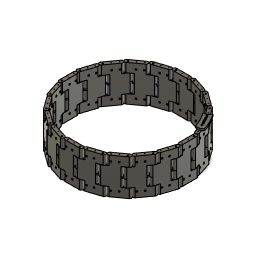
CAT_Wheel_Part v7 (Autodesk Fusion 360 design; units mm, degrees)
Autodesk Fusion 360 part; units mm, degrees
sketch "R_Part" plane through (0, 0, 0) normal (0, 1, 0) x (1, 0, 0)
  line L0 (75, 100) -> (0, 100)
  line L1 (0, 100) -> (0, 0)
  line L2 (150, 100) -> (150, 150)
  line L3 (150, 150) -> (75, 150)
  line L4 (75, 150) -> (75, 100)
  line L5 (150.000002, 100) -> (150.000002, 0)
  line L6 (150.000002, 0) -> (75, 0)
  line L7 (0, -50.000001) -> (75, -50)
  line L8 (75, -50) -> (75, 0)
  line L9 (0, 0) -> (0, -50.000001)
  dimension "d1" = 75
  dimension "d2" = 100
  dimension "d3" = 75
  dimension "d4" = 50
  dimension "d5" = 50
  dimension "d6" = 75.000002
  dimension "d7" = 150.000002
  constraint horizontal L0
  constraint vertical L1
  constraint coincident L1.end L9.start
  constraint vertical L2
  constraint horizontal L3
  constraint vertical L4
  constraint vertical L5
  constraint horizontal L6
  constraint horizontal L7
  constraint vertical L8
  constraint perpendicular L7 L9
  measures "d1" distance of L1.end L6.end
  measures "d2" distance of L1.end L0.end
  measures "d3" distance of L0.start L2.start
  measures "d4" distance of L0.start L3.end
  measures "d5" distance of L6.end L7.end
  measures "d7" distance of L1 L5
extrude "Extrude1" add sketch "R_Part" along normal blind 50 contours L0 L1 L2 L3 L4 L5 L6 L7 L8 L9 picked at (125.000001, 33.333333) makes body 1
extrude "Extrude2" cut 1 faces at (125.000001, 50, -33.333333) along direction (0, -1, 0) blind 20 on bodies 1 bodies 1
sketch "L_Part" plane through (0, 0, 0) normal (0, 1, 0) x (1, 0, 0)
  line L0 (-75, 0) -> (-150, 0)
  line L1 (-150, 0) -> (-150, 100)
  line L2 (-75, 100) -> (0, 100)
  line L3 (0, 100) -> (0, 0)
  line L4 (-75, 100) -> (-75, 150)
  line L5 (-75, 150) -> (-150, 150)
  line L6 (-150, 150) -> (-150, 100)
  line L7 (-75, 0) -> (-75, -50)
  line L8 (-75, -50) -> (0, -50)
  line L9 (0, -50) -> (0, 0)
  dimension "d13" = 150
  dimension "d14" = 100
  dimension "d15" = 75
  dimension "d16" = 50
  dimension "d17" = 75
  dimension "d18" = 50
  constraint horizontal L0
  constraint vertical L1
  constraint horizontal L2
  constraint vertical L3
  constraint coincident L3.end L9.end
  constraint vertical L4
  constraint horizontal L5
  constraint vertical L6
  constraint vertical L7
  constraint horizontal L8
  constraint vertical L9
  measures "d13" distance of L3.end L0.end
  measures "d14" distance of L3.end L2.end
  measures "d15" distance of L1.end L2.start
  measures "d16" distance of L1.end L5.end
  measures "d17" distance of L3.end L0.start
  measures "d18" distance of L3.end L8.end
sketch "Sketch3" plane through (0, 0, 50.000001) normal (0, 0, 1) x (1, 0, 0)
  line L0 (75, 30) -> (0, 30)
  line L1 (0, 30) -> (0, 0)
  line L2 (0, 0) -> (75, 0)
  line L3 (75, 0) -> (75, 30)
  line L4 (0, 0) -> (-10, 0)
  line L5 (-10, 0) -> (-10, 15)
  line L6 (-10, 15) -> (0, 15)
  line L7 (0, 15) -> (0, 0)
  line L8 (0, 15) -> (10, 15)
  line L9 (10, 15) -> (10, 30)
  line L10 (10, 30) -> (0, 30)
  line L11 (0, 30) -> (0, 15)
  dimension "d21" = 15
  dimension "d22" = 10
  dimension "d23" = 10
  constraint horizontal L4
  constraint vertical L5
  constraint horizontal L6
  constraint vertical L7
  constraint coincident L1.end L2.start
  constraint horizontal L8
  constraint vertical L9
  constraint horizontal L10
  constraint vertical L11
  measures "d21" distance of L1.end L6.end
  measures "d22" distance of L1.end L4.end
  measures "d23" distance of L6.end L8.end
extrude "Extrude4" add sketch "Sketch3" against normal blind 150 contours L1 L4 L5 L6 L7 picked at (-3.333334, 10) bodies 1
extrude "Extrude5" cut sketch "Sketch3" against normal blind 150 contours L0 L1 L8 L9 L10 L11 picked at (3.333333, 25) bodies 1
sketch "Sketch4" plane through (75, 0, 0) normal (1, 0, 0) x (0, 0, -1)
  line L0 (0, 30) -> (-50, 30)
  line L1 (-50, 30) -> (-50, 0)
  line L2 (-50, 0) -> (0, 0)
  line L3 (0, 0) -> (0, 30)
  circle A0 centre (-25, 15) radius 2.75
  dimension "d28" = 5.5
  measures "d28" diameter of A0
extrude "Extrude6" cut sketch "Sketch4" against normal blind 95 contours A0 picked at (-25.720575, 16.369678) bodies 1
sketch "Sketch5" plane through (75, 0, 0) normal (-1, 0, 0) x (0, 0, 1)
  line L0 (-100, 30) -> (-150, 30)
  line L1 (-150, 30) -> (-150, 0)
  line L2 (-150, 0) -> (-100, 0)
  line L3 (-100, 0) -> (-100, 30)
  circle A0 centre (-125, 15) radius 2.75
  dimension "d31" = 5.5
  measures "d31" diameter of A0
extrude "Extrude7" cut sketch "Sketch5" against normal blind 76 contours A0 picked at (-125.470371, 15.87372) bodies 1
sketch "Sketch6" plane through (150, 0, 0) normal (1, 0, 0) x (0, 0, -1)
  circle A0 centre (125, 15) radius 2.75
  line L0 (150, 30) -> (0, 30)
  line L1 (0, 30) -> (0, 0)
  line L2 (0, 0) -> (150, 0)
  line L3 (150, 0) -> (150, 30)
  line L4 (129.2, 17.424871) -> (125, 19.849742)
  line L5 (125, 19.849742) -> (120.8, 17.424871)
  line L6 (120.8, 17.424871) -> (120.8, 12.575129)
  line L7 (120.8, 12.575129) -> (125, 10.150258)
  line L8 (125, 10.150258) -> (129.2, 12.575129)
  line L9 (129.2, 12.575129) -> (129.2, 17.424871)
  point P0 (125, 15)
  dimension "d34" = 4.2
  constraint coincident P0 A0.centre
  measures "d34" distance of P0 L9
extrude "Extrude8" cut sketch "Sketch6" against normal blind 4.5 contours L4 L5 L6 L7 L8 L9 picked at (121.283333, 15) bodies 1
sketch "Sketch7" plane through (150, 0, 0) normal (1, 0, 0) x (0, 0, -1)
  line L0 (125, 19.849742) -> (129.2, 17.424871)
  line L1 (129.2, 17.424871) -> (129.2, 12.575129)
  line L2 (129.2, 12.575129) -> (125, 10.150258)
  line L3 (125, 10.150258) -> (120.8, 12.575129)
  line L4 (120.8, 12.575129) -> (120.8, 17.424871)
  line L5 (120.8, 17.424871) -> (125, 19.849742)
  line L6 (150, 30) -> (0, 30)
  line L7 (0, 30) -> (0, 0)
  line L8 (0, 0) -> (150, 0)
  line L9 (150, 0) -> (150, 30)
  line L10 (0, 0) -> (100.000001, 0)
  line L11 (100.000001, 0) -> (100.000001, 30)
  circle A0 centre (25, 15) radius 2.75
  circle A1 centre (75, 15) radius 2.75
  line L12 (-50.000001, 0) -> (99.999999, 0)
  point P0 (100, 0)
  dimension "d37" = 25
  dimension "d38" = 25
  dimension "d39" = 15
  dimension "d40" = 15
  dimension "d41" = 5.5
  dimension "d42" = 5.5
  constraint coincident L7.end L8.start
  constraint coincident L8 P0
  constraint perpendicular L7 L10
  constraint perpendicular L6 L11
  measures "d37" horizontal distance of L7.end A0.centre
  measures "d38" horizontal distance of A1.centre P0
  measures "d39" vertical distance of A1.centre P0
  measures "d40" distance of A0.centre L12
  measures "d41" diameter of A0
  measures "d42" diameter of A1
sketch "Sketch8" plane through (0, 30, 0) normal (0, 1, 0) x (-1, 0, 0)
  line L0 (-9.999999, -99.999999) -> (-10, 50.000001)
  line L1 (-10, 50.000001) -> (-75, 50)
  line L2 (-75, 50) -> (-75, 0)
  line L3 (-75, 0) -> (-150.000002, 0)
  line L4 (-150.000002, 0) -> (-150, -150)
  line L5 (-150, -150) -> (-75, -150)
  line L6 (-75, -150) -> (-75, -100)
  line L7 (-75, -100) -> (-9.999999, -99.999999)
  line L8 (-100, -30) -> (-110, -30)
  line L9 (-110, -30) -> (-110, -20)
  line L10 (-110, -20) -> (-100, -20)
  line L11 (-100, -20) -> (-100, -30)
  line L12 (-100.000002, -80) -> (-110.000002, -80)
  line L13 (-110.000002, -80) -> (-110.000002, -70)
  line L14 (-110.000002, -70) -> (-100.000002, -70)
  line L15 (-100.000002, -70) -> (-100.000002, -80)
  point P0 (-150, 0)
  point P1 (-150.000002, -100)
  dimension "d43" = 20
  dimension "d44" = 10
  dimension "d45" = 40
  dimension "d46" = 10
  dimension "d47" = 20
  dimension "d48" = 10
  dimension "d49" = 10
  dimension "d50" = 40
  constraint horizontal L8
  constraint vertical L9
  constraint horizontal L10
  constraint vertical L11
  constraint horizontal L12
  constraint vertical L13
  constraint horizontal L14
  constraint vertical L15
  measures "d43" vertical distance of L9.end P0
  measures "d44" distance of L8.end L9.end
  measures "d45" horizontal distance of L9.end P0
  measures "d46" distance of L9.end L10.end
extrude "Extrude9" cut sketch "Sketch8" against normal blind 54 contours L8 L9 L10 L11 picked at (-103.333333, -26.666667) bodies 1
extrude "Extrude10" cut sketch "Sketch8" against normal blind 51 contours L12 L13 L14 L15 picked at (-103.333336, -76.666667) bodies 1
extrude "Extrude11" cut sketch "Sketch7" against normal blind 44 contours A0 picked at (24.279425, 16.369678) bodies 1
extrude "Extrude12" cut sketch "Sketch7" against normal blind 48 contours A1 picked at (74.529629, 15.87372) bodies 1
sketch "Sketch9" plane through (110, 0, 0) normal (-1, 0, 0) x (0, 0, 1)
  circle A0 centre (-25, 15) radius 2.75
  line L0 (-30, 0) -> (-20, 0)
  line L1 (-20, 0) -> (-20, 30)
  line L2 (-20, 30) -> (-30, 30)
  line L3 (-30, 30) -> (-30, 0)
  line L4 (-20.9, 17.367136) -> (-25, 19.734272)
  line L5 (-25, 19.734272) -> (-29.1, 17.367136)
  line L6 (-29.1, 17.367136) -> (-29.1, 12.632864)
  line L7 (-29.1, 12.632864) -> (-25, 10.265728)
  line L8 (-25, 10.265728) -> (-20.9, 12.632864)
  line L9 (-20.9, 12.632864) -> (-20.9, 17.367136)
  point P0 (-25, 15)
  dimension "d59" = 4.1
  constraint coincident P0 A0.centre
  measures "d59" distance of P0 L9
extrude "Extrude13" cut sketch "Sketch9" against normal blind 4.5 contours L4 L5 L6 L7 L8 L9 picked at (-26.825, 18.160993) bodies 1
sketch "Sketch10" plane through (110.000002, 0, 0) normal (-1, 0, 0) x (0, 0, 1)
  circle A0 centre (-75, 15) radius 2.75
  line L0 (-80, 0) -> (-70, 0)
  line L1 (-70, 0) -> (-70, 30)
  line L2 (-70, 30) -> (-80, 30)
  line L3 (-80, 30) -> (-80, 0)
  line L4 (-70.9, 17.367136) -> (-75, 19.734272)
  line L5 (-75, 19.734272) -> (-79.1, 17.367136)
  line L6 (-79.1, 17.367136) -> (-79.1, 12.632864)
  line L7 (-79.1, 12.632864) -> (-75, 10.265728)
  line L8 (-75, 10.265728) -> (-70.9, 12.632864)
  line L9 (-70.9, 12.632864) -> (-70.9, 17.367136)
  point P0 (-75, 15)
  dimension "d62" = 4.1
  constraint coincident P0 A0.centre
  measures "d62" distance of P0 L9
extrude "Extrude14" cut sketch "Sketch10" against normal blind 4.5 contours L4 L5 L6 L7 L8 L9 picked at (-76.825, 18.160993) bodies 1
fillet "Fillet1" radius 15 1 edges at (42.5, 30, 50) on bodies 1
fillet "Fillet2" radius 15 1 edges at (32.5, 0, 50) on bodies 1
fillet "Fillet3" radius 15 1 edges at (112.500001, 30, 0) on bodies 1
fillet "Fillet4" radius 15 1 edges at (112.500001, 0, 0) on bodies 1
fillet "Fillet5" radius 15 1 edges at (42.5, 30, -100) on bodies 1
extrude "Extrude15" add 1 faces at (-6.666668, 5, -99.999999) along direction (-0.00000001, 0, -1) blind 1 on bodies 1 bodies 1
extrude "Extrude16" cut 1 faces at (0, 5, -100.666666) along direction (-1, 0, 0.00000001) blind 14 on bodies 1 bodies 1
fillet "Fillet6" radius 15 2 edges at (37.5, 0, -100) (-5, 0, -100) on bodies 1
fillet "Fillet7" radius 15 1 edges at (112.5, 30, -150) on bodies 1
fillet "Fillet8" radius 15 1 edges at (112.5, 0, -150) on bodies 1
copy_body "CopyPasteBodies2" bodies 1 makes body 2
move_body "Move1" bodies 2 to x (-1, 0, 0) y (0, -1, 0) z (0, 0, 1) at (0, 0, 0)
move_body "Move2" bodies 2 to x (1, 0, 0) y (0, 1, 0) z (0, 0, 1) at (0, 30, 0)
combine "Combine1" operation add target body 1 tool bodies 2
copy_body "Body->Comp1" bodies 1 removing the originals makes body 3 in component "R_PART"
sketch "Sketch11" plane through (0, 0, 0) normal (0, 1, 0) x (1, 0, 0)
  line L0 (-977.062727, 550) -> (0, 480) construction
  line L1 (-523.531364, 26.468636) -> (-453.531364, 1003.531364) construction
  circle A0 centre (-90.741812, 773.109327) radius 2.75
  circle A1 centre (-45.901699, 685.105652) radius 2.75
  arc A2 (-128.518801, 776.564437) -> (-79.977781, 811.831552) centre (-127.759701, 826.558675) ccw
  arc A3 (-65.311214, 652.512562) -> (-8.247823, 671.053582) centre (-49.140198, 699.825333) ccw
  arc A4 (-8.247823, 671.053582) -> (-79.977781, 811.831552) centre (-488.531364, 515) ccw
  arc A5 (-932.393702, 546.799764) -> (-43.531364, 515) centre (-488.531364, 515) ccw
  arc A6 (-65.311214, 652.512562) -> (-128.518801, 776.564437) centre (-488.531364, 515) ccw
  point P0 (-977.062727, 550)
  point P1 (0, 480)
  point P2 (-523.531364, 26.468636)
  point P3 (-453.531364, 1003.531364)
  dimension "d529" = 890
  dimension "d531" = 1010
  dimension "d534" = 50
  dimension "d535" = 50
  constraint coincident P1 L0.end
  constraint concentric A4 A5
  constraint concentric A5 A6
  measures "d529" diameter of A5
  measures "d531" diameter of A4
  measures "d534" radius of A2
  measures "d535" radius of A3
extrude "Extrude17" add sketch "Sketch11" along normal blind 15 separate body contours A2 A3 A4 A6 picked at (-60.509834, 741.800668) makes body 4
sketch "Sketch12" plane through (0, 15, 0) normal (0, 1, 0) x (-1, 0, 0)
  circle A0 centre (90.741812, -773.109327) radius 2.75
  circle A1 centre (45.901699, -685.105652) radius 2.75
  arc A2 (8.247823, -671.053582) -> (79.977781, -811.831552) centre (488.531364, -515) ccw
  arc A3 (128.518801, -776.564437) -> (79.977781, -811.831552) centre (127.759701, -826.558675) ccw
  arc A4 (65.311214, -652.512562) -> (128.518801, -776.564437) centre (488.531364, -515) ccw
  arc A5 (65.311214, -652.512562) -> (8.247823, -671.053582) centre (49.140198, -699.825333) ccw
  circle A6 centre (90.741812, -773.109327) radius 6
  circle A7 centre (45.901699, -685.105652) radius 6
  dimension "d538" = 12
  dimension "d539" = 12
  constraint concentric A0 A6
  constraint concentric A1 A7
  measures "d538" diameter of A7
  measures "d539" diameter of A6
extrude "Extrude18" cut sketch "Sketch12" against normal blind 6 contours A6 picked at (87.457196, -776.750014) bodies 4
extrude "Extrude19" cut sketch "Sketch12" against normal blind 6 contours A7 picked at (42.617084, -688.746339) bodies 4
sketch "Sketch13" plane through (0, 15, 0) normal (0, 1, 0) x (-1, 0, 0)
  circle A0 centre (45.901699, -685.105652) radius 6
  circle A1 centre (90.741812, -773.109327) radius 6
  arc A2 (8.247823, -671.053582) -> (79.977781, -811.831552) centre (488.531364, -515) ccw
  arc A3 (128.518801, -776.564437) -> (79.977781, -811.831552) centre (127.759701, -826.558675) ccw
  arc A4 (65.311214, -652.512562) -> (128.518801, -776.564437) centre (488.531364, -515) ccw
  arc A5 (65.311214, -652.512562) -> (8.247823, -671.053582) centre (49.140198, -699.825333) ccw
  line L0 (45.72209, -702.440421) -> (76.103896, -762.103906) construction
  line L1 (76.103896, -762.103906) -> (90.664492, -754.689367) construction
  line L2 (90.664492, -754.689367) -> (60.282686, -695.025883) construction
  line L3 (60.282686, -695.025883) -> (45.72209, -702.440421) construction
  text T0 "poohoenix" font "Impact" height 16.339717 align ink ink in box 0 x 0 at (45.72209, -702.440421) x (0.453774, -0.8911168) y (0.8911168, 0.453774) spacing 1 height is em
  constraint perpendicular L0 L1
  constraint parallel L0 L2
  constraint parallel L1 L3
extrude "Extrude20" cut sketch "Sketch13" against normal blind 1 text T0 bodies 4
copy_body "CopyPasteBodies3" bodies 4 makes body 5
move_body "Move3" bodies 5 to x (1, 0, 0) y (0, 1, 0) z (0, 0, 1) at (0, 150, 0)
sketch "Sketch14" plane through (-0.000001, 150, -0.000009) normal (0, 1, 0) x (-1, 0, 0)
  arc A0 (50.176871, -746.804289) -> (78.708567, -737.533779) centre (64.442719, -742.169034) ccw
  line L0 (78.708567, -737.533779) -> (41.626527, -623.406997)
  arc A1 (41.626527, -623.406997) -> (13.094832, -632.677506) centre (27.360679, -628.042252) ccw
  line L1 (13.094832, -632.677507) -> (50.176871, -746.804289)
  circle A2 centre (45.901699, -685.105643) radius 2.75
  circle A3 centre (30.450849, -637.552817) radius 2.75
  line L2 (65.964928, -731.159816) -> (64.95661, -735.90358)
  line L3 (64.95661, -735.90358) -> (60.344231, -737.402232)
  line L4 (60.344231, -737.402232) -> (56.74017, -734.157121)
  line L5 (56.74017, -734.157121) -> (57.748488, -729.413358)
  line L6 (57.748488, -729.413358) -> (62.360867, -727.914705)
  line L7 (62.360867, -727.914705) -> (65.964928, -731.159816)
  arc A4 (143.262934, -870.917966) -> (167.533444, -853.284409) centre (155.398189, -862.101188) ccw
  line L8 (167.533444, -853.284409) -> (96.999214, -756.20237)
  arc A5 (96.999214, -756.20237) -> (72.728704, -773.835927) centre (84.863959, -765.019148) ccw
  line L9 (72.728704, -773.835927) -> (143.262934, -870.917966)
  circle A6 centre (120.131074, -813.560168) radius 2.75
  circle A7 centre (90.741811, -773.109318) radius 2.75
  line L10 (153.443861, -851.160411) -> (153.950797, -855.983586)
  line L11 (153.950797, -855.983586) -> (150.027273, -858.834193)
  line L12 (150.027273, -858.834193) -> (145.596813, -856.861625)
  line L13 (145.596813, -856.861625) -> (145.089877, -852.03845)
  line L14 (145.089877, -852.03845) -> (149.013401, -849.187843)
  line L15 (149.013401, -849.187843) -> (153.443861, -851.160411)
  arc A8 (8.247823, -671.053573) -> (79.977781, -811.831544) centre (488.531363, -514.999991) ccw construction
  arc A9 (65.311214, -652.512554) -> (128.518801, -776.564428) centre (488.531363, -514.999991) ccw construction
  circle A10 centre (488.531363, -514.999991) radius 479.433992 construction
  circle A11 centre (61.352549, -732.658469) radius 2.75
  constraint concentric A9 A10
component "R_PART" placed x (0, 1, 0) y (-0.80901699, 0, -0.58778525) z (-0.58778525, 0, 0.80901699) at (-122.690451, 0, -187.397619)
component "R_PART" placed x (0, 1, 0) y (-0.95105652, 0, -0.30901699) z (-0.30901699, 0, 0.95105652) at (-39.361277, 0, -316.482681)
component "R_PART" placed x (0, 1, 0) y (-1, 0, 0) z (0, 0, 1) at (0, 0, -465)
component "R_PART" placed x (0, 1, 0) y (-0.95105652, 0, 0.30901699) z (0.30901699, 0, 0.95105652) at (-8.459577, 0, -618.411668)
component "R_PART" placed x (0, 1, 0) y (-0.58778525, 0, -0.80901699) z (-0.80901699, 0, 0.58778525) at (-241.830683, 0, -90.380562)
component "R_PART" placed x (0, 1, 0) y (-0.30901699, 0, -0.95105652) z (-0.95105652, 0, 0.30901699) at (-385.119696, 0, -34.928214)
component "R_PART" placed x (0, 1, 0) y (0, 0, -1) z (-1, 0, 0) at (-538.531364, 0, -26.468636)
component "R_PART" placed x (0, 1, 0) y (0.30901699, 0, -0.95105652) z (-0.95105652, 0, -0.30901699) at (-687.048683, 0, -65.829913)
component "R_PART" placed x (0, 1, 0) y (-0.80901699, 0, 0.58778525) z (0.58778525, 0, 0.80901699) at (-63.911926, 0, -761.700681)
component "R_PART" placed x (0, 1, 0) y (-0.58778525, 0, 0.80901699) z (0.80901699, 0, 0.58778525) at (-160.928983, 0, -880.840913)
component "R_PART" placed x (0, 1, 0) y (0.58778525, 0, -0.80901699) z (-0.80901699, 0, -0.58778525) at (-816.133744, 0, -149.159087)
component "R_PART" placed x (0, 1, 0) y (-0.30901699, 0, 0.95105652) z (0.95105652, 0, 0.30901699) at (-290.014044, 0, -964.170087)
component "R_PART" placed x (0, 1, 0) y (0.80901699, 0, -0.58778525) z (-0.58778525, 0, -0.80901699) at (-913.150802, 0, -268.299319)
component "R_PART" placed x (0, 1, 0) y (0, 0, 1) z (1, 0, 0) at (-438.531364, 0, -1003.531364)
component "R_PART" placed x (0, 1, 0) y (0.95105652, 0, -0.30901699) z (-0.30901699, 0, -0.95105652) at (-968.60315, 0, -411.588332)
component "R_PART" placed x (0, 1, 0) y (0.30901699, 0, 0.95105652) z (0.95105652, 0, -0.30901699) at (-591.943031, 0, -995.071786)
component "R_PART" placed x (0, 1, 0) y (0.58778525, 0, 0.80901699) z (0.80901699, 0, -0.58778525) at (-735.232045, 0, -939.619438)
component "R_PART" placed x (0, 1, 0) y (0.80901699, 0, 0.58778525) z (0.58778525, 0, -0.80901699) at (-854.372276, 0, -842.602381)
component "R_PART" placed x (0, 1, 0) y (0.95105652, 0, 0.30901699) z (0.30901699, 0, -0.95105652) at (-937.701451, 0, -713.517319)
component "R_PART" placed x (0, 1, 0) y (1, 0, 0) z (0, 0, -1) at (-977.062727, 0, -565)
hidden bodies 4
named bodies: "R_PART", "L_PART"
